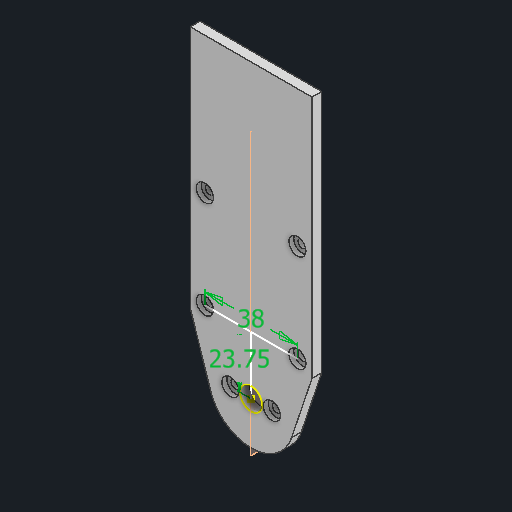
# Autodesk Inventor part: plate_base
Saved by Autodesk Inventor 2026 (Build 300175000, 175)
## iProperties
Created: 2026-08-17
Part Number: plate_base
Material: Generic
Document SubType Name: Modeling
Designer: imcle
Density: 1 g/cm^3
Appearance: Default
Author: imcle
Autodesk Inventor part; units mm, degrees
ref_plane "YZ Plane" through (0, 0, 0) normal (1, 0, 0) x (0, 1, 0)
ref_plane "XZ Plane" through (0, 0, 0) normal (0, 1, 0) x (-1, 0, 0)
ref_plane "XY Plane" through (0, 0, 0) normal (0, 0, 1) x (1, 0, 0)
sketch "Sketch1" plane through (0, 0, 0) normal (0, 0, 1) x (1, 0, 0)
  circle A0 centre (0, 0) radius 4.5
  line L0 (-8.5, 0) -> (8.5, 0)
  circle A1 centre (8.5, 0) radius 1.75
  circle A2 centre (-8.5, 0) radius 1.75
  arc A3 (-16.6079, -5.5163) -> (16.6079, -5.5163) centre (0, 0) ccw
  line L1 (0, 0) -> (0, 19.75)
  line L2 (-25, 19.75) -> (25, 19.75)
  line L3 (-25, 19.75) -> (-16.6079, -5.5163)
  line L4 (25, 19.75) -> (16.6079, -5.5163)
  line L5 (-25, 19.75) -> (25, 19.75)
  line L6 (25, 19.75) -> (25, 119.75)
  line L7 (25, 119.75) -> (-25, 119.75)
  line L8 (-25, 119.75) -> (-25, 19.75)
  point P0 (25, 19.75)
  dimension "d0" = 9
  dimension "d1" = 17
  dimension "d2" = 3.5
  dimension "d3" = 3.5
  dimension "d4" = 35
  dimension "d5" = 19.75
  dimension "d6" = 50
  dimension "d7" = 50
  dimension "d8" = 100
  constraints: 18 end point, 4 centre point, 4 coincident, 3 horizontal, 2 midpoint, 2 parallel, 2 point on circle, 2 tangent, 1 perpendicular, 1 vertical
  measures "d0" diameter of A0
  measures "d1" distance of L0.start L0.end
  measures "d2" diameter of A1
  measures "d3" diameter of A2
  measures "d4" diameter of A3
  measures "d5" distance of L1.start L1.end
  measures "d6" distance of L2.start L2.end
  measures "d7" distance of L7.end L6.end
  measures "d8" distance of L5.end L6.end
extrude "Extrusion1" add sketch "Sketch1" along normal blind 4
sketch "Sketch2" plane through (0, 0, 4) normal (0, 0, 1) x (1, 0, 0)
  circle A0 centre (8.5, 0) radius 1.75 projected
  circle A1 centre (-8.5, 0) radius 1.75 projected
  circle A2 centre (8.5, 0) radius 3.5
  point P0 (0, 0)
  dimension "d12" = 7
  constraints: 1 centre point
  measures "d12" diameter of A2
ref_plane "Work Plane1" through (0, 19.75, 0) normal (1, 0, 0) x (0, 0, -1)
extrude "Extrusion2" cut sketch "Sketch2" against normal blind 2 contours A2
mirror "Mirror1" about plane through (0, 19.75, 0) normal (1, 0, 0) of "Extrusion2"
sketch "Sketch3" plane through (0, 0, 4) normal (0, 0, 1) x (1, 0, 0)
  circle A0 centre (0, 0) radius 4.5 projected
  line L0 (0, 0) -> (0, 23.75)
  line L1 (-19, 23.75) -> (19, 23.75)
  dimension "d15" = 23.75
  dimension "d16" = 38
  constraints: 4 end point, 1 horizontal, 1 midpoint, 1 vertical
  measures "d15" distance of L0.start L0.end
  measures "d16" distance of L1.start L1.end
sketch "Sketch4" plane through (0, 0, 4) normal (0, 0, 1) x (1, 0, 0)
  circle A0 centre (-19, 23.75) radius 1.75
  circle A1 centre (-19, 23.75) radius 3.5
  point P0 (0, 0)
  dimension "d17" = 3.5
  dimension "d18" = 7
  constraints: 2 centre point, 2 coincident
  measures "d17" diameter of A0
  measures "d18" diameter of A1
extrude "Extrusion3" cut sketch "Sketch4" against normal up to surface (4 mm away) contours A0
extrude "Extrusion4" cut sketch "Sketch4" against normal blind 2
mirror "Mirror2" about plane through (0, 19.75, 0) normal (1, 0, 0) of "Extrusion4", "Extrusion3"
pattern_linear "Rectangular Pattern1" count 2 spacing 40 along (0, 1, 0) count 2 spacing 38 along (1, 0, 0) of "Extrusion4", "Extrusion3"
body "Solid1"
